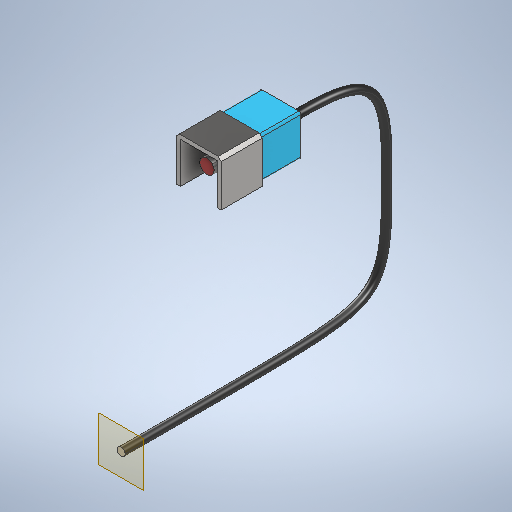
# Autodesk Inventor part: sensor
Saved by Autodesk Inventor 2025 (Build 290162000, 162)
## iProperties
Created: 2024-10-02
Part Number: sensor
Material: Generic
Document SubType Name: Modeling
Designer: DMIADX
Density: 1 g/cm^3
Appearance: Default
Author: DMIADX
Autodesk Inventor part; units mm, degrees
ref_plane "YZ Plane" through (0, 0, 0) normal (1, 0, 0) x (0, 1, 0)
ref_plane "XZ Plane" through (0, 0, 0) normal (0, 1, 0) x (-1, 0, 0)
ref_plane "XY Plane" through (0, 0, 0) normal (0, 0, 1) x (1, 0, 0)
sketch "Sketch1" plane through (0, 0, 0) normal (0, 0, 1) x (1, 0, 0)
  line L0 (10, -10) -> (-10, -10)
  line L1 (-10, -10) -> (-10, 10)
  line L2 (-10, 10) -> (10, 10)
  line L3 (10, 10) -> (10, -10)
  line L4 (10, -10) -> (-10, 10) construction
  line L5 (-10, -10) -> (10, 10) construction
  point P0 (0, 0)
  dimension "d0" = 20
  dimension "d1" = 20
  constraints: 12 end point, 2 midpoint, 2 parallel, 1 horizontal, 1 perpendicular
  measures "d0" distance of L1.end L2.end
  measures "d1" distance of L0.end L1.end
extrude "Extrusion1" add sketch "Sketch1" along normal blind 20
sketch "Sketch2" plane through (0, 0, 20) normal (0, 0, 1) x (1, 0, 0)
  line L0 (10, 10) -> (-10, 10) projected
  line L1 (-10, 10) -> (-10, -10) projected
  line L2 (-10, -10) -> (10, -10) projected
  line L3 (10, -10) -> (10, 10) projected
  line L4 (-11, 11) -> (11, 11)
  line L5 (11, 11) -> (11, -11)
  line L6 (11, -11) -> (-11, -11)
  line L7 (-11, -11) -> (-11, 11)
  line L8 (-9, 9) -> (9, 9)
  line L9 (9, 9) -> (9, -11)
  line L10 (9, -9) -> (-9, -9)
  line L11 (-9, -11) -> (-9, 9)
  point P0 (0, 0)
  dimension "d4" = 1
  dimension "d5" = 1
  constraints: 16 end point, 4 point on line, 3 other
  measures "d4" distance between parallel lines of L0 L4
  measures "d5" distance between parallel lines of L0 L8
extrude "Extrusion2" add sketch "Sketch2" along normal blind 20 contours L3 L2 L9 L8 L11 L1 L0 | L0 L1 L2 L11 L6 L7 L4 L5 L9 L3
chamfer "Chamfer1" distance 1.5 angle 45 2 edges at (11, 11, 30) (-11, 11, 30)
fillet "Fillet1" radius 1 4 edges at (10, 10, 10) (-10, 10, 10) (10, -10, 10) (-10, -10, 10)
sketch "Sketch3" plane through (0, 0, 20) normal (0, 0, 1) x (1, 0, 0)
  circle A0 centre (0, 0) radius 3.5
  dimension "d12" = 7
  constraints: 1 centre point, 1 coincident
  measures "d12" diameter of A0
extrude "Extrusion3" add sketch "Sketch3" along normal blind 16 and the other way blind 22
ref_plane "Work Plane1" through (0, -100, 78) normal (0, 0, 1) x (1, 0, 0)
sketch "Sketch4" plane through (0, -100, 78) normal (0, 0, 1) x (1, 0, 0)
  circle A0 centre (0, 0) radius 2
  point P0 (0, 100)
  dimension "d17" = 4
  constraints: 1 centre point
  measures "d17" diameter of A0
sketch3d "3D Sketch1"
  spline S0 degree 4 poles (0, 0, -2) (0, 0, -22) (0, 0, -52) (0, -40, -52) (0, -60, -52) (0, -100, -52) (0, -100, -22) (0, -100, 48) (0, -100, 78) knots 1 1 1 1 1 2 3 4 5 6 6 6 6 6
  dimension "d20" = 40
  dimension "d21" = 70
  dimension "d22" = 100
sweep "Sweep1" add profiles "Sketch4" path "3D Sketch1"
body "Solid1"
